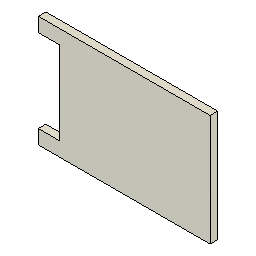
SchubplatteDisplaygehäuse (Autodesk Fusion 360 design; units mm, degrees)
Autodesk Fusion 360 part; units mm, degrees
sketch "Skizze1" plane through (0, 0, 0) normal (0, 0, 1) x (1, 0, 0)
  line L0 (0, 0) -> (0, 29.5)
  line L1 (0, 29.5) -> (-45.5, 29.5)
  line L2 (-45.5, 29.5) -> (-45.5, 25.75)
  line L3 (-45.5, 25.75) -> (-40, 25.75)
  line L4 (-40, 25.75) -> (-40, 3.75)
  line L5 (-40, 3.75) -> (-45.5, 3.75)
  line L6 (-45.5, 3.75) -> (-45.5, 0)
  line L7 (-45.5, 0) -> (0, 0)
  dimension "d1" = 29.5
  dimension "d2" = 45.5
  dimension "d3" = 22
  dimension "d4" = 3.75
  dimension "d7" = 45.5
  constraint coincident L0.start L7.end
  constraint vertical L0
  constraint perpendicular L0 L1
  constraint perpendicular L1 L2
  constraint perpendicular L2 L3
  constraint perpendicular L3 L4
  constraint perpendicular L4 L5
  constraint perpendicular L5 L6
  constraint perpendicular L0 L7
  measures "d1" distance of L0.start L0.end
  measures "d2" distance of L0.end L1.end
  measures "d3" distance of L3.end L4.end
  measures "d4" distance of L1.end L2.end
  measures "d7" distance of L6.end L0.start
extrude "Extrusion1" add sketch "Skizze1" along normal blind 2
